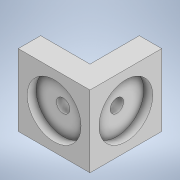
# Autodesk Inventor part: MountingBracket_2
Saved by Autodesk Inventor 2020 (Build 240168000, 168)
## iProperties
Created: 2022-02-07
Part Number: MountingBracket_2
Material: Generic
Document SubType Name: Modeling
Designer: danie
Density: 1 g/cm^3
Appearance: Default
Author: danie
Autodesk Inventor part; units mm, degrees
ref_plane "YZ Plane" through (0, 0, 0) normal (1, 0, 0) x (0, 1, 0)
ref_plane "XZ Plane" through (0, 0, 0) normal (0, 1, 0) x (-1, 0, 0)
ref_plane "XY Plane" through (0, 0, 0) normal (0, 0, 1) x (1, 0, 0)
sketch "Sketch1" plane through (0, 0, 0) normal (0, 1, 0) x (-1, 0, 0)
  line L0 (0, 0) -> (-25.4, 0)
  line L1 (-25.4, 0) -> (-25.4, -25.4)
  line L2 (-25.4, -25.4) -> (0, -25.4)
  line L3 (0, -25.4) -> (0, 0)
  line L4 (0, 0) -> (-25.4, -25.4) construction
  line L5 (-25.4, 0) -> (0, -25.4) construction
  circle A0 centre (-12.7, -12.7) radius 9.525
  dimension "d0" = 25.4
  dimension "d1" = 25.4
  dimension "d3" = 19.05
  constraints: 12 end point, 2 parallel, 1 centre point, 1 horizontal, 1 perpendicular
  measures "d0" distance of L2.end L1.end
  measures "d1" distance of L1.end L0.end
  measures "d3" diameter of A0
extrude "Extrusion1" add sketch "Sketch1" along normal blind 3.175
sketch "Sketch2" plane through (0, 3.175, 0) normal (0, 1, 0) x (1, 0, 0)
  line L0 (25.4, 25.4) -> (0, 25.4) projected
  line L1 (0, 0) -> (25.4, 0)
  line L2 (25.4, 0) -> (25.4, 25.4)
  line L3 (25.4, 25.4) -> (0, 25.4)
  line L4 (0, 25.4) -> (0, 0)
  line L5 (0, 25.4) -> (0, 0) construction
  line L6 (0, 0) -> (25.4, 25.4) construction
  line L7 (0, 25.4) -> (25.4, 0) construction
  circle A0 centre (12.7, 12.7) radius 2.3812
  dimension "d6" = 4.7625
  constraints: 12 end point, 2 parallel, 1 centre point, 1 horizontal, 1 midpoint, 1 perpendicular
  measures "d6" diameter of A0
extrude "Extrusion2" add sketch "Sketch2" along normal blind 4.7625
sketch "Sketch4" plane through (0, 0, 0) normal (0, 0, 1) x (1, 0, 0)
  line L0 (0, 0) -> (0, 7.9375) projected
  line L1 (0, 0) -> (25.4, 0)
  line L2 (25.4, 0) -> (25.4, 25.4)
  line L3 (25.4, 25.4) -> (0, 25.4)
  line L4 (0, 25.4) -> (0, 0)
  line L5 (0, 25.4) -> (25.4, 0) construction
  line L6 (25.4, 25.4) -> (0, 0) construction
  circle A0 centre (12.7, 12.7) radius 9.525
  dimension "d13" = 25.4
  dimension "d14" = 25.4
  dimension "d15" = 19.05
  constraints: 12 end point, 2 parallel, 1 centre point, 1 horizontal, 1 midpoint, 1 perpendicular
  measures "d13" distance of L3.end L2.end
  measures "d14" distance of L2.end L1.end
  measures "d15" diameter of A0
extrude "Extrusion4" add sketch "Sketch4" against normal blind 3.175
sketch "Sketch5" plane through (0, 0, 0) normal (0, 0, 1) x (1, 0, 0)
  line L0 (0, 0) -> (0, 25.4) construction
  line L1 (0, 0) -> (25.4, 0) construction
  line L2 (0, 25.4) -> (25.4, 0) construction
  line L3 (0, 25.4) -> (25.4, 25.4) construction
  line L4 (25.4, 0) -> (25.4, 25.4) construction
  line L5 (0, 0) -> (0, 7.9375) construction
  line L6 (25.4, 25.4) -> (0, 0) construction
  circle A0 centre (12.7, 12.7) radius 9.525
  dimension "d18" = 19.05
  constraints: 6 end point, 2 perpendicular, 1 centre point, 1 midpoint
  measures "d18" diameter of A0
extrude "Extrusion5" cut sketch "Sketch5" against normal blind 3.175
sketch "Sketch6" plane through (0, 0, -3.175) normal (0, 0, -1) x (-1, 0, 0)
  line L0 (-25.4, 0) -> (-25.4, 25.4) projected
  line L1 (-25.4, 25.4) -> (0, 25.4)
  line L2 (0, 25.4) -> (0, 0)
  line L3 (0, 0) -> (-25.4, 0)
  line L4 (-25.4, 0) -> (-25.4, 25.4)
  line L5 (0, 0) -> (0, 25.4) construction
  line L6 (-25.4, 25.4) -> (0, 0) construction
  line L7 (0, 0) -> (0, 25.4) construction
  line L8 (0, 25.4) -> (-25.4, 0) construction
  circle A0 centre (-12.7, 12.7) radius 2.3813
  dimension "d21" = 4.7625
  constraints: 14 end point, 3 perpendicular, 2 parallel, 1 centre point, 1 horizontal, 1 midpoint
  measures "d21" diameter of A0
extrude "Extrusion6" add sketch "Sketch6" along normal blind 4.7625
sketch "Sketch7" plane through (25.4, 0, 0) normal (1, 0, 0) x (0, 0, -1)
  line L0 (0, 25.4) -> (7.9375, 25.4) projected
  line L1 (25.4, 0) -> (25.4, 7.9375) projected
  line L2 (0, 25.4) -> (25.4, 25.4)
  line L3 (25.4, 25.4) -> (25.4, 0)
  line L4 (25.4, 0) -> (0, 0)
  line L5 (0, 0) -> (0, 25.4)
  line L6 (0, 25.4) -> (25.4, 0) construction
  line L7 (25.4, 25.4) -> (0, 0) construction
  circle A0 centre (12.7, 12.7) radius 9.525
  dimension "d24" = 19.05
  constraints: 12 end point, 2 parallel, 2 perpendicular, 1 centre point, 1 horizontal, 1 midpoint
  measures "d24" diameter of A0
extrude "Extrusion7" add sketch "Sketch7" against normal blind 3.175
sketch "Sketch8" plane through (25.4, 0, 0) normal (1, 0, 0) x (0, 0, -1)
  line L0 (0, 0) -> (0, 25.4) construction
  line L1 (0, 0) -> (25.4, 0) construction
  line L2 (0, 25.4) -> (25.4, 0) construction
  line L3 (25.4, 0) -> (25.4, 25.4) construction
  line L4 (25.4, 25.4) -> (0, 0) construction
  circle A0 centre (12.7, 12.7) radius 9.525
  dimension "d27" = 19.05
  constraints: 6 end point, 1 centre point, 1 midpoint, 1 perpendicular
  measures "d27" diameter of A0
extrude "Extrusion8" cut sketch "Sketch8" against normal blind 3.175
sketch "Sketch9" plane through (22.225, 0, 0) normal (-1, 0, 0) x (0, 0, 1)
  line L0 (-25.4, 25.4) -> (-25.4, 7.9375) projected
  line L1 (-25.4, 25.4) -> (0, 25.4)
  line L2 (0, 25.4) -> (0, 0)
  line L3 (0, 0) -> (-25.4, 0)
  line L4 (-25.4, 0) -> (-25.4, 25.4)
  line L5 (-25.4, 0) -> (0, 0) construction
  line L6 (-25.4, 25.4) -> (0, 0) construction
  line L7 (0, 0) -> (0, 25.4) construction
  line L8 (0, 25.4) -> (-25.4, 0) construction
  circle A0 centre (-12.7, 12.7) radius 2.3813
  dimension "d30" = 4.7625
  constraints: 14 end point, 3 equal length, 1 centre point, 1 horizontal, 1 midpoint, 1 perpendicular
  measures "d30" diameter of A0
extrude "Extrusion9" add sketch "Sketch9" along normal blind 4.7625
sketch "Sketch10" plane through (0, 0, 0) normal (0, -1, 0) x (1, 0, 0)
  line L0 (0, -25.4) -> (0, -7.9375) projected
  line L1 (25.4, 0) -> (0, 0) projected
  line L2 (0, -25.4) -> (25.4, -25.4)
  line L3 (25.4, -25.4) -> (25.4, 0)
  line L4 (25.4, 0) -> (0, 0)
  line L5 (0, 0) -> (0, -25.4)
  line L6 (17.4625, -25.4) -> (0, -25.4) construction
  line L7 (25.4, 0) -> (25.4, -25.4) construction
  line L8 (0, -25.4) -> (25.4, 0) construction
  line L9 (25.4, 0) -> (0, 0) construction
  line L10 (0, -25.4) -> (0, 0) construction
  line L11 (0, 0) -> (25.4, -25.4) construction
  circle A0 centre (12.7, -12.7) radius 9.525
  dimension "d33" = 19.05
  constraints: 14 end point, 2 parallel, 2 perpendicular, 1 centre point, 1 horizontal, 1 midpoint
  measures "d33" diameter of A0
extrude "Extrusion10" cut sketch "Sketch10" against normal blind 3.175 contours A0
sketch "Sketch11" plane through (0, 0, 0) normal (0, 0, 1) x (1, 0, 0)
  line L0 (0, 7.9375) -> (0, 25.4) construction
  line L1 (25.4, 0) -> (25.4, 25.4) construction
  line L2 (0, 25.4) -> (25.4, 0) construction
  line L3 (25.4, 0) -> (25.4, 25.4) construction
  line L4 (25.4, 25.4) -> (0, 0) construction
  circle A0 centre (12.7, 12.7) radius 9.525
  dimension "d36" = 19.05
  constraints: 6 end point, 1 centre point, 1 collinear, 1 midpoint, 1 perpendicular
  measures "d36" diameter of A0
extrude "Extrusion11" cut sketch "Sketch11" against normal blind 3.175
body "Solid1"
